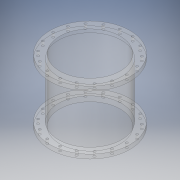
# Autodesk Inventor part: Reaktor
Saved by Autodesk Inventor 2017 (Build 210142000, 142)
## iProperties
Part Number: Reaktor
Material: PET-Kunststoff
Document SubType Name: Modeling
Designer: Benjamin
Density: 1.541 g/cm^3
Appearance: Polycarbonat - klar
Author: Benjamin
Autodesk Inventor part; units mm, degrees
ref_plane "YZ Plane" through (0, 0, 0) normal (1, 0, 0) x (0, 1, 0)
ref_plane "XZ Plane" through (0, 0, 0) normal (0, 1, 0) x (-1, 0, 0)
ref_plane "XY Plane" through (0, 0, 0) normal (0, 0, 1) x (1, 0, 0)
sketch "Skizze1" plane through (0, 0, 0) normal (1, 0, 0) x (0, 1, 0)
  line L0 (190, 0) -> (144, 0)
  line L1 (144, 0) -> (144, 300)
  line L2 (144, 300) -> (190, 300)
  line L3 (190, 300) -> (190, 280)
  line L4 (190, 0) -> (190, 20)
  line L5 (163.8, 300) -> (190, 300)
  line L6 (0, 0) -> (0, 300)
  line L7 (190, 280) -> (150, 280)
  line L8 (150, 280) -> (150, 20)
  line L9 (150, 20) -> (190, 20)
  dimension "d0" = 46
  dimension "d1" = 300
  dimension "d2" = 46
  dimension "d3" = 20
  dimension "d9" = 300
  dimension "d48" = 40
  constraints: 20 end point, 6 perpendicular, 2 horizontal, 1 point on line, 1 vertical
  measures "d0" distance of L0.start L0.end
  measures "d1" distance of L0.end L1.end
  measures "d2" distance of L2.end L1.end
  measures "d3" distance of L2.end L3.end
  measures "d9" distance of L6.start L6.end
  measures "d48" distance of L3.end L7.end
revolve "Umdrehung1" add sketch "Skizze1" angle 360 about axis through (0, 0, 0) along (0, 0, 1)
sketch "Skizze3" plane through (0, 0, 0) normal (0, 0, -1) x (-1, 0, 0)
  circle A0 centre (175, 0) radius 5.5 projected
  point P0 (0, 0)
  constraints: 1 coincident
hole "Bohrung2" at (-175, 0, 0) direction (0, 0, 1) diameter 11 depth 25 tip angle 118
pattern_circular "Runde Anordnung2" count 18 over 360 about axis through (0, 0, 150) along (0, 0, -1) of "Bohrung2"
sketch "Skizze12" plane through (0, 0, 300) normal (0, 0, 1) x (1, 0, 0)
  point P0 (0, 0)
  point P1 (-175, 0)
  dimension "d51" = 175
  measures "d51" distance of point (0, 0) point (-175, 0)
hole "Bohrung3" at (-175, 0, 300) direction (0, 0, -1) diameter 11 depth 30 tip angle 118
pattern_circular "Runde Anordnung3" count 18 over 360 about axis through (0, 0, -10) along (0, 0, 1) of "Bohrung3"
